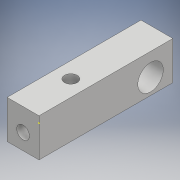
# Autodesk Inventor part: SupportCodeuse
Saved by Autodesk Inventor 2017 SP1 (Build 210196100, 196)
## iProperties
Part Number: SupportCodeuse
Material: Générique
Document SubType Name: Modeling
Designer: Sylvain
Density: 1 g/cm^3
Appearance: Par défaut
Author: Sylvain
## iProperties of the stored document SupportCodeuse_Impression 3D.ipt
Part Number: SupportCodeuse_Impression 3D
Material: Générique
Document SubType Name: Modeling
Designer: Sylvain
Density: 1 g/cm^3
Appearance: Par défaut
Author: Sylvain
Autodesk Inventor part; units mm, degrees
ref_plane "YZ Plane" through (0, 0, 0) normal (1, 0, 0) x (0, 1, 0)
ref_plane "XZ Plane" through (0, 0, 0) normal (0, 1, 0) x (-1, 0, 0)
ref_plane "XY Plane" through (0, 0, 0) normal (0, 0, 1) x (1, 0, 0)
sketch "Esquisse1" plane through (0, 0, 0) normal (1, 0, 0) x (0, 1, 0)
  line L0 (0, 0) -> (40, 0)
  line L1 (40, 0) -> (40, -10)
  line L2 (40, -10) -> (0, -10)
  line L3 (0, -10) -> (0, 0)
  dimension "d0" = 40
  dimension "d1" = 10
  constraints: 8 end point, 2 parallel, 1 horizontal, 1 perpendicular
  measures "d0" distance between parallel lines of L3 L1
  measures "d1" distance between parallel lines of L2 L0
extrude "Extrusion1" add sketch "Esquisse1" along normal blind 10
sketch "Esquisse2" plane through (10, 0, 0) normal (1, 0, 0) x (0, 0, -1)
  line L0 (10, 40) -> (0, 40) projected
  line L1 (0, 40) -> (0, 0) projected
  point P0 (5, 35)
  dimension "d4" = 5
  dimension "d5" = 5
  measures "d4" distance from line of L0 point (5, 35)
  measures "d5" distance from line of L1 point (5, 35)
hole "Perçage1" at (10, 35, -5) direction (-1, 0, 0) diameter 8 depth 10 tip angle 118
sketch "Esquisse3" plane through (0, 0, 0) normal (0, 0, 1) x (1, 0, 0)
  line L0 (0, 40) -> (0, 0) projected
  line L1 (10, 0) -> (10, 40) projected
  line L2 (0, 40) -> (10, 40)
  line L3 (10, 40) -> (10, 0)
  line L4 (10, 0) -> (0, 0)
  line L5 (0, 0) -> (0, 40)
  constraints: 8 end point, 2 parallel, 1 horizontal, 1 perpendicular
extrude "Extrusion2" add sketch "Esquisse3" along normal blind 2
sketch "Esquisse4" plane through (0, 40, -10) normal (0, 1, 0) x (1, 0, 0)
  line L0 (0, 0) -> (0, -12) projected
  line L1 (0, 0) -> (10, 0) projected
  line L2 (0, -12) -> (10, -12)
  line L3 (10, -12) -> (10, 0)
  line L4 (10, 0) -> (0, 0)
  line L5 (0, 0) -> (0, -12)
  point P0 (0, -10)
  constraints: 8 end point, 2 parallel, 1 horizontal, 1 perpendicular
extrude "Extrusion3" add sketch "Esquisse4" along normal blind 2
sketch "Esquisse5" plane through (10, 0, 0) normal (1, 0, 0) x (0, 0, -1)
  point P0 (0, 0)
sketch "Esquisse6" plane through (0, 0, -10) normal (0, -1, 0) x (1, 0, 0)
  line L0 (0, 0) -> (10, 0) projected
  line L1 (0, 0) -> (0, 12) projected
  point P0 (0, 10)
  point P1 (5, 5)
  dimension "d17" = 5
  dimension "d18" = 5
  measures "d17" distance from line of L0 point (5, 5)
  measures "d18" distance from line of L1 point (5, 5)
hole "Perçage2" at (5, 0, -5) direction (0, 1, 0) diameter 4 depth 6 tip angle 118
sketch "Esquisse7" plane through (10, 0, -10) normal (0, 0, -1) x (-1, 0, 0)
  line L0 (10, 0) -> (0, 0) projected
  line L1 (0, 0) -> (0, 42) projected
  point P0 (5, 15)
  dimension "d26" = 15
  dimension "d27" = 5
  measures "d26" distance from line of L0 point (5, 15)
  measures "d27" distance from line of L1 point (5, 15)
hole "Perçage3" at (5, 15, -10) direction (0, 0, 1) diameter 4 depth 12 tip angle 118
